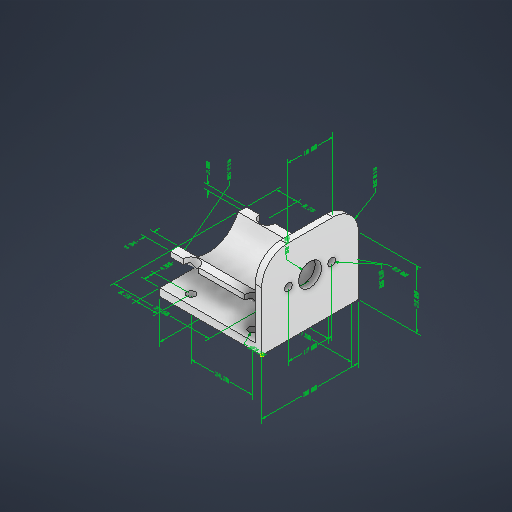
# Autodesk Inventor part: Base_nueva
Saved by Autodesk Inventor 2026.2 (Build 302298000, 298)
## iProperties
Created: 2026-01-30
Part Number: Base_nueva
Material: Genérico
Document SubType Name: Sheet Metal
Designer: yahir
Density: 1 g/cm^3
Sheet Metal Rule: Por defecto_mm
Appearance: Valor por defecto
Author: yahir
## iProperties of the stored document Base_nueva_3DPrint.ipt
Created: 2026-02-02
Part Number: Base_nueva_3DPrint
Material: Genérico
Document SubType Name: Modeling
Designer: yahir
Density: 1 g/cm^3
Appearance: Valor por defecto
Author: yahir
Autodesk Inventor part; units mm, degrees
ref_plane "YZ Plane" through (0, 0, 0) normal (1, 0, 0) x (0, 1, 0)
ref_plane "XZ Plane" through (0, 0, 0) normal (0, 1, 0) x (-1, 0, 0)
ref_plane "XY Plane" through (0, 0, 0) normal (0, 0, 1) x (1, 0, 0)
sketch "Boceto1" plane through (0, 0, 0) normal (0, 1, 0) x (-1, 0, 0)
  point P0 (0, 0)
sketch "Boceto2" plane through (0, 0, 0) normal (0, 1, 0) x (-1, 0, 0)
  line L0 (0, 0) -> (40, 0)
  line L1 (40, 0) -> (40, -38)
  line L2 (40, -38) -> (0, -38)
  line L3 (0, -38) -> (0, 0)
  dimension "d0" = 40
  dimension "d1" = 38
  constraints: 8 end point, 2 parallel, 1 horizontal, 1 perpendicular
  measures "d0" distance of L1.end L2.end
  measures "d1" distance of L0.end L1.end
extrude "Extrusión1" add sketch "Boceto2" along normal blind 3
sketch "Boceto3" plane through (0, 3, 0) normal (0, 1, 0) x (1, 0, 0)
  line L0 (0, 0) -> (0, 38) projected
  line L1 (0, 0) -> (-2.5, 0)
  line L2 (-40, 0) -> (0, 0) projected
  line L3 (-2.5, 0) -> (-2.5, 38)
  line L4 (-2.5, 38) -> (0, 38)
  line L5 (0, 38) -> (0, 0)
  dimension "d4" = 2.5
  dimension "d5" = 38
  constraints: 8 end point, 3 perpendicular, 1 point on line
  measures "d4" distance of L0.start L1.end
  measures "d5" distance of L1.end L3.end
extrude "Extrusión2" add sketch "Boceto3" along normal blind 30
sketch "Boceto4" plane through (0, 0, 0) normal (1, 0, 0) x (0, 0, -1)
  line L0 (0, 0) -> (38, 0) projected
  circle A0 centre (19, 18) radius 4.5
  line L1 (19, 0) -> (19, 18)
  dimension "d9" = 9
  dimension "d21" = 18
  constraints: 2 end point, 1 centre point, 1 midpoint, 1 vertical
  measures "d9" diameter of A0
  measures "d21" distance of L1.start L1.end
extrude "Extrusión3" cut sketch "Boceto4" against normal blind 30
sketch "Boceto5" plane through (0, 0, 0) normal (1, 0, 0) x (0, 0, -1)
  circle A0 centre (19, 18) radius 4.5 projected
  line L0 (19, 18) -> (27.5, 18)
  line L1 (19, 18) -> (10.5, 18)
  circle A1 centre (10.5, 18) radius 1.5
  circle A2 centre (27.5, 18) radius 1.5
  point P0 (0, 0)
  dimension "d12" = 8.5
  dimension "d13" = 8.5
  dimension "d14" = 3
  dimension "d15" = 3
  constraints: 4 end point, 2 centre point, 2 coincident, 2 horizontal
  measures "d12" distance of L0.start L0.end
  measures "d13" distance of L0.start L1.end
  measures "d14" diameter of A1
  measures "d15" diameter of A2
extrude "Extrusión4" cut sketch "Boceto5" against normal blind 8.5 contours A1 | A2
fillet "Empalme1" radius 10 1 edges at (-1.25, 33, 0)
fillet "Empalme2" radius 10 1 edges at (-1.25, 33, -38)
sketch "Boceto6" plane through (-2.5, 3, -38) normal (-1, 0, 0) x (0, 0, 1)
  circle A0 centre (19, 15) radius 4.5 projected
  arc A1 (7.3381, 10.5) -> (30.6619, 10.5) centre (19, 15) ccw
  line L0 (30.6619, 10.5) -> (34, 10.5)
  circle A2 centre (19, 15) radius 4.5 projected
  line L1 (4, 10.5) -> (7.3381, 10.5)
  line L2 (34, 8.5) -> (31.9615, 8.5)
  arc A3 (6.0385, 8.5) -> (31.9615, 8.5) centre (19, 15) ccw
  line L3 (6.0385, 8.5) -> (4, 8.5)
  line L4 (4, 10.5) -> (4, 8.5)
  line L5 (0, 0) -> (0, 20) projected
  line L6 (34, 10.5) -> (34, 8.5)
  line L7 (38, 0) -> (38, 20) projected
  point P0 (38, -3)
  dimension "d20" = 25
  dimension "d27" = 2
  constraints: 12 end point, 4 point on circle, 2 centre point, 2 collinear, 2 horizontal, 2 vertical, 1 coincident, 1 point on line, 5 other
  measures "d20" diameter of A1
  measures "d27" radial gap between concentric circles of A1 A3
extrude "Extrusión5" add sketch "Boceto6" along normal blind 37.5 contours A1 L0 L6 L2 A3 L3 L4 L1
sketch "Boceto9" plane through (0, 0, 0) normal (0, -1, 0) x (1, 0, 0)
  line L0 (0, 0) -> (0, -38) projected
  line L1 (0, -38) -> (0, -19)
  line L2 (0, -19) -> (-7.55, -19)
  line L3 (-7.55, -19) -> (-7.55, -4)
  line L4 (-7.55, -19) -> (-7.55, -34)
  circle A0 centre (-7.55, -4) radius 1.6
  circle A1 centre (-7.55, -34) radius 1.6
  line L5 (-7.55, -4) -> (-31.75, -4)
  line L6 (-2.5, -4) -> (-40, -4) projected
  line L7 (-31.75, -4) -> (-31.75, -34)
  circle A2 centre (-31.75, -4) radius 1.6
  circle A3 centre (-31.75, -34) radius 1.6
  dimension "d33" = 19
  dimension "d34" = 7.55
  dimension "d35" = 15
  dimension "d37" = 15
  dimension "d38" = 3.2
  dimension "d39" = 3.2
  dimension "d41" = 24.2
  dimension "d42" = 30
  dimension "d43" = 3.2
  dimension "d44" = 3.2
  constraints: 12 end point, 4 centre point, 3 coincident, 2 vertical, 1 horizontal, 1 midpoint, 1 perpendicular, 1 point on line
  measures "d33" distance of L0.end L1.end
  measures "d34" distance of L1.end L2.end
  measures "d35" distance of L2.end L3.end
  measures "d37" distance of L2.end L4.end
  measures "d38" diameter of A0
  measures "d39" diameter of A1
  measures "d41" distance of L5.start L5.end
  measures "d42" distance of L5.end L7.end
  measures "d43" diameter of A2
  measures "d44" diameter of A3
extrude "Extrusión6" cut sketch "Boceto9" against normal blind 3
sketch "Boceto10" plane through (0, 3, 0) normal (0, 1, 0) x (1, 0, 0)
  circle A0 centre (-31.75, 4) radius 1.6 projected
  circle A1 centre (-31.75, 4) radius 3
  circle A2 centre (-7.55, 4) radius 1.6 projected
  circle A3 centre (-7.55, 4) radius 3
  circle A4 centre (-31.75, 34) radius 1.6 projected
  circle A5 centre (-31.75, 34) radius 3
  line L0 (-2.5, 34) -> (-40, 34) projected
  circle A6 centre (-7.55, 34) radius 3
  point P0 (0, 0)
  dimension "d58" = 6
  dimension "d59" = 6
  dimension "d60" = 6
  dimension "d61" = 6
  constraints: 4 centre point, 3 coincident, 1 point on line
  measures "d58" diameter of A1
  measures "d59" diameter of A3
  measures "d60" diameter of A5
  measures "d61" diameter of A6
extrude "Extrusión7" cut sketch "Boceto10" along normal blind 20 contours A0 | A1 | A2 | A3 | L0 A4 | L0 A5 A4 | A4 L0 A5 | A4 L0 | A6 L0 | L0 A6
sketch "Boceto11" plane through (-40, 0, -38) normal (-1, 0, 0) x (0, 0, 1)
  line L0 (0, 3) -> (38, 3) projected
  arc A0 (6.0385, 11.5) -> (31.9615, 11.5) centre (19, 18) ccw projected
  line L1 (19, 4.5) -> (24.2915, 4.5)
  line L2 (19, 4.5) -> (13.7085, 4.5)
  line L3 (13.7085, 4.5) -> (13.7085, 3)
  line L4 (24.2915, 4.5) -> (24.2915, 3)
  line L5 (13.7085, 3) -> (24.2915, 3)
  point P0 (38, 0)
  constraints: 10 end point, 2 point on circle, 2 point on line, 1 collinear, 1 horizontal, 1 perpendicular, 1 vertical
extrude "Extrusión8" add sketch "Boceto11" against normal blind 40
equation "\"d16\" = d12"
equation "\"Radio_pliegue\" = Grosor"
equation "\"Anchura_desahogo_plegado\" = Grosor"
equation "\"Profundidad_desahogo_plegado\" = 0.5 * Grosor"
equation "\"Tamaño_destalonado\" = 4 * Grosor"
equation "\"Remanente_mínimo\" = 2 * Grosor"
equation "\"Radiodetransición\" = Radio_pliegue"
equation "\"Tamaño_de_radio_de_Jacobi\" = Radio_pliegue"
equation "\"TamañoSeparación\" = Grosor"
equation "\"Grosor\" = 0.5"
